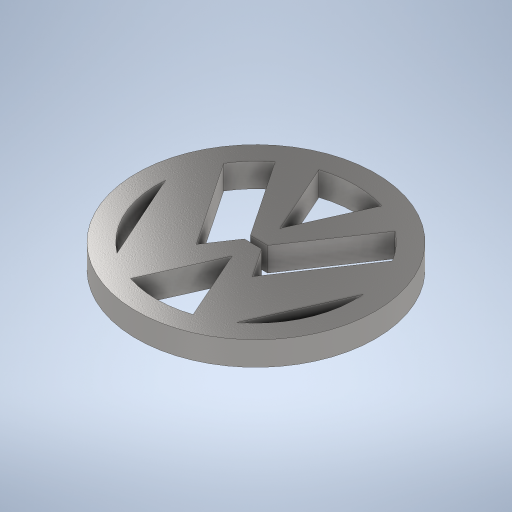
# Autodesk Inventor part: VW
Saved by Autodesk Inventor 2024 (Build 280153000, 153)
## iProperties
Created: 2024-02-01
Part Number: VW
Material: Stahl, galvanisiert
Document SubType Name: Modeling
Designer: ffogue
Density: 7.85 g/cm^3
Appearance: Galvanisiert
Author: ffogue
Autodesk Inventor part; units mm, degrees
ref_plane "XZ Plane" through (0, 0, 0) normal (0, 1, 0) x (-1, 0, 0)
ref_plane "XY Plane" through (0, 0, 0) normal (0, 0, 1) x (1, 0, 0)
sketch "Skizze2" plane through (0, 0, 0) normal (0, 0, 1) x (1, 0, 0)
  circle A0 centre (0, 0) radius 50
  circle A1 centre (0, 0) radius 41.5 construction
  dimension "d12" = 100
  dimension "d13" = 83
  constraints: 2 centre point, 2 coincident
  measures "d12" diameter of A0
  measures "d13" diameter of A1
extrude "Extrusion3" add sketch "Skizze2" against normal blind 10
sketch "Skizze3" plane through (0, 0, 0) normal (0, 0, 1) x (1, 0, 0)
  circle A0 centre (0, 0) radius 50 projected
  line L0 (0, 50) -> (0, -50) construction
  line L1 (-50, 0) -> (50, 0) construction
  line L2 (0, -10) -> (-13.0826, -39.384)
  line L3 (0, -10) -> (13.0826, -39.384)
  circle A1 centre (0, 0) radius 41.5 construction
  arc A2 (-13.0826, -39.384) -> (13.0826, -39.384) centre (0, 0) ccw
  dimension "d16" = 48
  dimension "d17" = 10
  constraints: 8 end point, 6 point on circle, 2 midpoint, 1 centre point, 1 perpendicular, 1 point on line, 1 symmetric about line, 1 vertical, 3 other
  measures "d16" angle of L3 L2
  measures "d17" distance of point (0, 0) L2.start
extrude "Extrusion4" cut sketch "Skizze3" against normal up to surface (10 mm away) contours L3 A2 L2
pattern_circular "Runde Anordnung1" count 2 over 360 about axis through (0, 0, 0) along (0, 0, -1) of "Extrusion4"
sketch "Skizze4" plane through (0, 0, 0) normal (0, 0, 1) x (1, 0, 0)
  line L0 (-50, 0) -> (50, 0) construction
  line L1 (0, 50) -> (0, -50) construction
  line L2 (-3.6024, 1.25) -> (3.6024, 1.25)
  line L3 (-3.6024, -1.25) -> (3.6024, -1.25)
  line L4 (3.6024, 1.25) -> (25.0677, 33.0736)
  circle A0 centre (0, 0) radius 41.5 construction
  line L5 (13.0826, 39.384) -> (0, 10) projected
  line L6 (3.6024, -1.25) -> (11.6965, -13.25)
  line L7 (11.6965, -13.25) -> (35.325, 21.7807)
  line L8 (0, -10) -> (13.0826, -39.384) projected
  arc A1 (35.325, 21.7807) -> (25.0677, 33.0736) centre (0, 0) ccw
  line L9 (-3.6024, 1.25) -> (-25.0677, 33.0736)
  line L10 (0, 10) -> (-13.0826, 39.384) projected
  line L11 (-3.6024, -1.25) -> (-11.6965, -13.25)
  line L12 (-11.6965, -13.25) -> (-35.325, 21.7807)
  arc A2 (-25.0677, 33.0736) -> (-35.325, 21.7807) centre (0, 0) ccw
  line L13 (-13.0826, -39.384) -> (0, -10) projected
  dimension "d23" = 2.5
  dimension "d30" = 12
  dimension "d31" = 10
  dimension "d32" = 10
  dimension "d33" = 10
  dimension "d34" = 10
  constraints: 16 end point, 4 point on circle, 2 centre point, 2 horizontal, 2 parallel, 2 symmetric about line, 1 horizontal alignment, 1 vertical alignment, 8 other
  measures "d23" distance between parallel lines of L3 L2
  measures "d30" vertical distance of L11.end L3.start
  measures "d31" angle of L10 L9
  measures "d32" angle of L4 L5
  measures "d33" angle of L13 L11
  measures "d34" angle of L6 L8
extrude "Extrusion5" cut sketch "Skizze4" against normal up to surface (10 mm away)
sketch "Skizze5" plane through (0, 0, 0) normal (0, 0, 1) x (1, 0, 0)
  circle A0 centre (0, 0) radius 41.5 construction
  line L0 (0, 50) -> (0, -50) construction
  line L1 (-50, 0) -> (50, 0) construction
  line L2 (-11.6965, -13.25) -> (-35.325, 21.7807) projected
  line L3 (-41.352, 3.5016) -> (-25.0677, -33.0736)
  line L4 (-13.4789, -15.8926) -> (-28.8614, -38.698) construction
  line L5 (-3.6024, -1.25) -> (-11.6965, -13.25) projected
  arc A1 (-41.352, 3.5016) -> (-25.0677, -33.0736) centre (0, 0) ccw
  point P0 (-33.2098, -14.786)
  dimension "d41" = 10
  constraints: 5 point on circle, 4 end point, 2 point on line, 1 centre point, 1 collinear, 1 concentric, 1 midpoint
  measures "d41" angle of L2 L3
extrude "Extrusion6" cut sketch "Skizze5" against normal up to surface (10 mm away)
ref_plane "Arbeitsebene1" through (0, 0, 0) normal (1, 0, 0) x (0, 1, 0)
mirror "Spiegeln1" about plane through (0, 0, 0) normal (1, 0, 0) of "Extrusion6"
equation "\"d32\" = d31"
